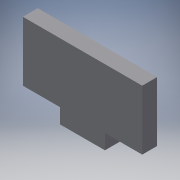
# Autodesk Inventor part: Part7
Saved by Autodesk Inventor 2018 (Build 220112000, 112)
## iProperties
Created: 2018-05-22
Part Number: Part7
Material: Generic
Document SubType Name: Modeling
Designer: Administrator
Density: 1 g/cm^3
Appearance: Default
Author: Administrator
Autodesk Inventor part; units mm, degrees
ref_plane "YZ Plane" through (0, 0, 0) normal (1, 0, 0) x (0, 1, 0)
ref_plane "XZ Plane" through (0, 0, 0) normal (0, 1, 0) x (-1, 0, 0)
ref_plane "XY Plane" through (0, 0, 0) normal (0, 0, 1) x (1, 0, 0)
sketch "Sketch1" plane through (0, 0, 0) normal (0, 0, 1) x (1, 0, 0)
  line L0 (14.8808, 25.4) -> (-10.5192, 25.4)
  line L1 (-10.5192, 25.4) -> (-10.5192, 0)
  line L2 (-10.5192, 0) -> (14.8808, 0)
  line L3 (14.8808, 0) -> (14.8808, 25.4)
  line L4 (6.9433, 0) -> (-2.5817, 0)
  line L5 (-2.5817, 0) -> (-2.5817, -3.175)
  line L6 (-2.5817, -3.175) -> (6.9433, -3.175)
  line L7 (6.9433, -3.175) -> (6.9433, 0)
  point P0 (0, 0)
  dimension "d0" = 25.4
  dimension "d1" = 25.4
  dimension "d2" = 7.9375
  dimension "d3" = 7.9375
  dimension "d4" = 3.175
  constraints: 16 end point, 4 parallel, 2 horizontal, 2 perpendicular, 1 point on line
  measures "d0" distance between parallel lines of L1 L3
  measures "d1" distance between parallel lines of L0 L2
  measures "d2" distance between parallel lines of L3 L7
  measures "d3" distance between parallel lines of L1 L5
  measures "d4" distance between parallel lines of L2 L6
extrude "Extrusion1" add sketch "Sketch1" along normal blind 3.175
body "Solid1"
